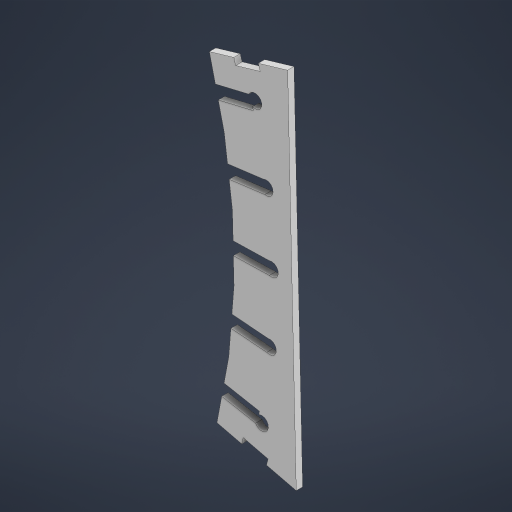
# Autodesk Inventor part: Back Plate
Saved by Autodesk Inventor 2023 (Build 270158000, 158)
## iProperties
Created: 2022-06-13
Part Number: Back Plate
Material: Generic
Document SubType Name: Modeling
Designer: FizzyApple12
Density: 1 g/cm^3
Appearance: Default
Author: FizzyApple12
Autodesk Inventor part; units mm, degrees
ref_plane "YZ Plane" through (0, 0, 0) normal (1, 0, 0) x (0, 1, 0)
ref_plane "XZ Plane" through (0, 0, 0) normal (0, 1, 0) x (-1, 0, 0)
ref_plane "XY Plane" through (0, 0, 0) normal (0, 0, 1) x (1, 0, 0)
ref_plane "Work Plane2" through (388.0538, -686.9281, 216.8066) normal (0, 0, 1) x (-0.9917416, -0.1282521, 0)
sketch "Sketch3" plane through (388.0538, -686.9281, 216.8066) normal (0, 0, 1) x (-0.9917416, -0.1282521, 0)
  line L0 (4.3583, 15.8159) -> (10.8533, 46.3726) construction
  line L1 (1.0044, -15.8113) -> (4.2698, 15.2569) construction
  line L2 (1.0044, -15.8113) -> (4.2698, 15.2569) construction
  line L3 (0.9748, -47.6157) -> (0.9748, -16.3764) construction
  line L4 (0.9748, -47.6157) -> (0.9748, -16.3764) construction
  line L5 (4.2698, -79.2491) -> (1.0044, -48.1809) construction
  line L6 (4.2698, -79.2491) -> (1.0044, -48.1809) construction
  line L7 (10.9998, 46.9192) -> (20.6533, 76.6296) construction
  line L8 (4.3583, 15.8159) -> (10.8533, 46.3726) construction
  line L9 (10.9998, 46.9192) -> (20.6533, 76.6296) construction
  line L10 (20.6533, 76.6296) -> (-103.8397, 124.4179) construction
  line L11 (-117.8064, 81.4327) -> (10.9998, 46.9192) construction
  line L12 (10.8533, 46.3726) -> (-117.9529, 80.8861) construction
  line L13 (-127.3499, 36.6764) -> (4.3583, 15.8159) construction
  line L14 (4.2698, 15.2569) -> (-127.4385, 36.1175) construction
  line L15 (0.9748, -16.3764) -> (-132.1925, -9.3974) construction
  line L16 (-132.1629, -8.8323) -> (1.0044, -15.8113) construction
  line L17 (1.0044, -48.1809) -> (-132.1629, -55.1599) construction
  line L18 (-132.1925, -54.5947) -> (0.9748, -47.6157) construction
  line L19 (-127.4385, -100.1096) -> (4.2698, -79.2491) construction
  line L20 (19.0965, 77.2271) -> (9.3891, 47.3508)
  line L21 (9.3891, 47.3508) -> (9.2426, 46.8041)
  line L22 (9.2426, 46.8041) -> (2.7113, 16.0767)
  line L23 (2.7113, 16.0767) -> (2.6228, 15.5178)
  line L24 (2.6228, 15.5178) -> (-0.6609, -15.724)
  line L25 (-0.6609, -15.724) -> (-0.6905, -16.2891)
  line L26 (-0.6905, -16.2891) -> (-0.6905, -47.703)
  line L27 (-0.6905, -47.703) -> (-0.6609, -48.2681)
  line L28 (-0.6609, -48.2681) -> (2.6228, -79.5099)
  line L29 (2.6228, -79.5099) -> (-36.3059, -75.4184)
  line L30 (-36.3059, -75.4184) -> (-19.8322, 81.3187)
  line L31 (-19.8322, 81.3187) -> (19.0965, 77.2271)
  line L32 (-127.4385, 36.1175) -> (-129.1369, 19.9578) construction
  point P0 (296.7492, -731.0239)
  dimension "d32" = 1.6652
  dimension "d33" = 1.6652
  dimension "d34" = 1.6652
  dimension "d35" = 1.6652
  dimension "d36" = 1.6652
  dimension "d37" = 29.21
  constraints: 24 end point, 10 point on line, 8 parallel, 1 perpendicular
  measures "d32" distance between parallel lines of L1 L24
  measures "d33" distance between parallel lines of L22 L0
  measures "d34" distance between parallel lines of L20 L7
  measures "d35" distance between parallel lines of L26 L3
  measures "d36" distance between parallel lines of L6 L28
  measures "d37" distance between parallel lines of L30 L24
extrude "Extrusion3" add sketch "Sketch3" along normal blind 3.175
sketch "Sketch5" plane through (388.0538, -686.9281, 219.9816) normal (0, 0, 1) x (0.9917416, 0.1282521, 0)
  line L0 (-19.0965, -77.2271) -> (19.8322, -81.3187) projected
  line L1 (-19.0965, -77.2271) -> (-19.1979, -77.4913)
  line L2 (-19.1979, -77.4913) -> (-7.3415, -82.0426)
  line L3 (4.515, -86.5938) -> (18.7052, -92.0409)
  line L4 (19.8322, -81.3187) -> (36.3059, 75.4184) projected
  line L5 (19.8322, -81.3187) -> (18.7052, -92.0409)
  line L6 (-18.0601, -74.5272) -> (-19.1979, -77.4913) construction
  line L7 (36.3059, 75.4184) -> (37.4328, 86.1406)
  line L8 (37.4328, 86.1406) -> (22.4202, 83.7628)
  line L9 (9.8766, 81.7761) -> (-2.6671, 79.7894)
  line L10 (36.3059, 75.4184) -> (-2.6228, 79.5099) projected
  line L11 (-2.6671, 79.7894) -> (-2.6228, 79.5099)
  line L12 (-2.6671, 79.7894) -> (-2.1704, 76.6535) construction
  line L13 (1.5509, -85.456) -> (-4.3773, -83.1804) projected
  line L14 (2.6887, -82.4919) -> (1.5509, -85.456) projected
  line L15 (-3.2395, -80.2163) -> (2.6887, -82.4919) projected
  line L16 (-3.2395, -80.2163) -> (-4.3773, -83.1804) projected
  line L17 (19.781, 80.1302) -> (13.5092, 79.1369) projected
  line L18 (19.2843, 83.2662) -> (19.781, 80.1302) projected
  line L19 (13.0125, 82.2728) -> (19.2843, 83.2662) projected
  line L20 (13.0125, 82.2728) -> (13.5092, 79.1369) projected
  line L21 (13.5092, 79.1369) -> (13.0125, 82.2728) projected
  line L22 (13.0125, 82.2728) -> (9.8766, 81.7761) projected
  line L23 (9.8766, 81.7761) -> (10.3733, 78.6402) projected
  line L24 (13.5092, 79.1369) -> (10.3733, 78.6402) projected
  line L25 (19.2843, 83.2662) -> (19.781, 80.1302) projected
  line L26 (22.9169, 80.6269) -> (19.781, 80.1302) projected
  line L27 (22.4202, 83.7628) -> (22.9169, 80.6269) projected
  line L28 (22.4202, 83.7628) -> (19.2843, 83.2662) projected
  line L29 (2.6887, -82.4919) -> (1.5509, -85.456) projected
  line L30 (4.515, -86.5938) -> (1.5509, -85.456) projected
  line L31 (5.6528, -83.6297) -> (4.515, -86.5938) projected
  line L32 (5.6528, -83.6297) -> (2.6887, -82.4919) projected
  line L33 (-4.3773, -83.1804) -> (-3.2395, -80.2163) projected
  line L34 (-3.2395, -80.2163) -> (-6.2036, -79.0785) projected
  line L35 (-6.2036, -79.0785) -> (-7.3415, -82.0426) projected
  line L36 (-4.3773, -83.1804) -> (-7.3415, -82.0426) projected
  point P0 (-296.7492, 731.0239)
  point P1 (2.6887, -82.4919)
  point P2 (19.781, 80.1302)
  point P3 (13.5092, 79.1369)
  constraints: 16 end point, 4 collinear, 3 parallel, 1 perpendicular
extrude "Extrusion4" add sketch "Sketch5" against normal blind 3.175 contours L0 L5 L3 L31 L32 L15 L34 L35 L2 L1 | L10 L11 L9 L23 L24 L17 L26 L27 L8 L7
sketch "Sketch6" plane through (388.0538, -686.9281, 219.9816) normal (0, 0, 1) x (0.9917416, 0.1282521, 0)
  line L0 (16.6451, 79.6336) -> (18.6318, 67.0899) construction
  line L1 (-0.2754, -81.3541) -> (4.2759, -69.4976) construction
  line L2 (18.7052, -92.0409) -> (37.4328, 86.1406) construction
  line L3 (28.069, -2.9502) -> (17.9647, -1.8882) construction
  line L4 (-6.2036, -79.0785) -> (5.6528, -83.6297) construction
  line L5 (22.9169, 80.6269) -> (10.3733, 78.6402) construction
  point P0 (-296.7492, 731.0239)
  dimension "d23" = 12.7
  dimension "d24" = 12.7
  dimension "d55" = 10.16
  constraints: 6 end point, 3 coincident, 3 midpoint, 3 perpendicular
  measures "d23" distance of L0.start L0.end
  measures "d24" distance of L1.start L1.end
  measures "d55" distance from line of L3.end L2
hole "Hole2" at (401.2076, -755.3034, 219.9816) at (397.9274, -618.0027, 219.9816) at (406.1123, -686.4967, 219.9816) direction (0, 0, -1) diameter 6.7564 depth 13.6144 clearance for "Flat Head Machine Screw (82)" size "1/4" standard "Ansi Unified Screw Threads"
sketch "Sketch7" plane through (388.0538, -686.9281, 219.9816) normal (0, 0, 1) x (0.9917416, 0.1282521, 0)
  line L0 (0.6609, 15.724) -> (-2.6228, -15.5178) construction
  line L1 (-0.981, 0.1031) -> (5.3342, -0.5607) construction
  line L2 (-6.4804, -2.5114) -> (16.4852, -4.9251)
  line L3 (16.4852, -4.9251) -> (17.1489, 1.3901)
  line L4 (17.1489, 1.3901) -> (-5.8167, 3.8038)
  line L5 (-5.8167, 3.8038) -> (-6.4804, -2.5114)
  line L6 (-6.4804, -2.5114) -> (17.1489, 1.3901) construction
  line L7 (16.4852, -4.9251) -> (-5.8167, 3.8038) construction
  circle A0 centre (17.9647, -1.8882) radius 3.3782 construction
  line L8 (10.8679, -38.2669) -> (-11.7196, -33.4657)
  line L9 (-11.7196, -33.4657) -> (-10.3994, -27.2545)
  line L10 (-10.3994, -27.2545) -> (12.1881, -32.0556)
  line L11 (12.1881, -32.0556) -> (10.8679, -38.2669)
  line L12 (10.8679, -38.2669) -> (-10.3994, -27.2545) construction
  line L13 (-11.7196, -33.4657) -> (12.1881, -32.0556) construction
  line L14 (-20.1657, -63.7029) -> (1.7962, -70.8387)
  line L15 (1.7962, -70.8387) -> (3.7585, -64.7995)
  line L16 (3.7585, -64.7995) -> (-18.2034, -57.6637)
  line L17 (-18.2034, -57.6637) -> (-20.1657, -63.7029)
  line L18 (-20.1657, -63.7029) -> (3.7585, -64.7995) construction
  line L19 (1.7962, -70.8387) -> (-18.2034, -57.6637) construction
  line L20 (18.5865, 35.1711) -> (-4.5056, 35.1711)
  line L21 (-4.5056, 35.1711) -> (-4.5056, 28.8211)
  line L22 (-4.5056, 28.8211) -> (18.5865, 28.8211)
  line L23 (18.5865, 28.8211) -> (18.5865, 35.1711)
  line L24 (18.5865, 35.1711) -> (-4.5056, 28.8211) construction
  line L25 (-4.5056, 35.1711) -> (18.5865, 28.8211) construction
  line L26 (-6.4804, 66.5035) -> (-5.8167, 60.1883)
  line L27 (-5.8167, 60.1883) -> (17.1489, 62.6021)
  line L28 (17.1489, 62.6021) -> (16.4852, 68.9173)
  line L29 (16.4852, 68.9173) -> (-6.4804, 66.5035)
  line L30 (-6.4804, 66.5035) -> (17.1489, 62.6021) construction
  line L31 (-5.8167, 60.1883) -> (16.4852, 68.9173) construction
  line L32 (-9.3891, -47.3508) -> (-19.0965, -77.2271) construction
  line L33 (-14.2428, -62.289) -> (-8.2036, -64.2512) construction
  line L34 (-2.7113, -16.0767) -> (-9.2426, -46.8041) construction
  line L35 (-5.977, -31.4404) -> (0.2343, -32.7607) construction
  line L36 (0.6905, 47.703) -> (0.6905, 16.2891) construction
  line L37 (0.6905, 31.9961) -> (7.0405, 31.9961) construction
  line L38 (-2.6228, 79.5099) -> (0.6609, 48.2681) construction
  line L39 (-0.981, 63.889) -> (5.3342, 64.5528) construction
  point P0 (-296.7492, 731.0239)
  point P1 (0.2343, -32.7607)
  point P2 (-8.2036, -64.2512)
  point P3 (5.3342, 64.5528)
  dimension "d38" = 6.35
  dimension "d39" = 6.35
  dimension "d40" = 23.0921
  dimension "d41" = 6.35
  dimension "d42" = 6.35
  dimension "d43" = 6.35
  dimension "d44" = 6.35
  dimension "d45" = 6.35
  dimension "d46" = 6.35
  dimension "d47" = 6.35
  dimension "d48" = 6.35
  dimension "d49" = 23.0921
  dimension "d50" = 23.0921
  dimension "d51" = 23.0921
  dimension "d52" = 23.0921
  constraints: 70 end point, 19 midpoint, 15 perpendicular, 10 parallel, 2 other
  measures "d38" distance of L1.start L1.end
  measures "d39" distance of L3.end L2.end
  measures "d40" distance between parallel lines of L3 L5
  measures "d41" distance of L33.end L33.start
  measures "d42" distance of L35.end L35.start
  measures "d43" distance of L37.end L37.start
  measures "d44" distance of L39.end L39.start
  measures "d45" distance between parallel lines of L14 L16
  measures "d46" distance between parallel lines of L22 L20
  measures "d47" distance between parallel lines of L8 L10
  measures "d48" distance between parallel lines of L29 L27
  measures "d49" distance between parallel lines of L28 L26
  measures "d50" distance between parallel lines of L21 L23
  measures "d51" distance between parallel lines of L9 L11
  measures "d52" distance between parallel lines of L17 L15
extrude "Extrusion5" cut sketch "Sketch7" against normal blind 3.175
sketch "Sketch8" plane through (388.0538, -686.9281, 219.9816) normal (0, 0, 1) x (0.9917416, 0.1282521, 0)
  line L0 (0.6609, 15.724) -> (-0.6491, 3.2607) construction
  arc A0 (16.4852, -4.9251) -> (17.1489, 1.3901) centre (17.9647, -1.8882) ccw construction
  line L1 (18.5865, 35.1711) -> (18.5865, 28.8211) construction
  line L2 (18.5865, 31.9961) -> (19.7405, 31.9961) construction
  line L3 (0.6905, 47.703) -> (0.6905, 35.1711) construction
  line L4 (10.8679, -38.2669) -> (12.1881, -32.0556) construction
  line L5 (11.528, -35.1612) -> (12.6567, -35.4012) construction
  line L6 (-2.7113, -16.0767) -> (-5.3169, -28.3348) construction
  point P0 (-296.7492, 731.0239)
  dimension "d56" = 19.05
  dimension "d57" = 19.05
  dimension "d58" = 19.05
  constraints: 4 end point, 2 coincident, 2 midpoint, 2 perpendicular
  measures "d56" distance from line of L0 A0.centre
  measures "d57" distance from line of L3 L2.end
  measures "d58" distance from line of L6 point (12.657, -35.401)
hole "Hole3" at (403.5277, -652.6645, 219.9816) at (405.1463, -720.4137, 219.9816) direction (0, 0, -1) diameter 6.7564 depth 13.6144 clearance for "Flat Head Machine Screw (82)" size "1/4" standard "Ansi Unified Screw Threads"
equation "\"d33\" = d32"
equation "\"d34\" = d32"
equation "\"d36\" = d32"
equation "\"d45\" = d39"
equation "\"d46\" = d39"
equation "\"d47\" = d39"
equation "\"d48\" = d39"
equation "\"d49\" = d40"
equation "\"d50\" = d40"
equation "\"d51\" = d40"
equation "\"d52\" = d40"
equation "\"d57\" = d56"
equation "\"d58\" = d56"
body "Solid3"
